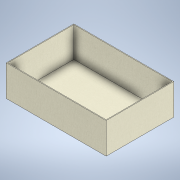
# Autodesk Inventor part: Box_Base
Saved by Autodesk Inventor 2021 (Build 250183000, 183)
## iProperties
Created: 2023-03-16
Part Number: Box_Base
Material: Paper
Document SubType Name: Modeling
Designer: Bradley
Density: 0.93 g/cm^3
Appearance: Cardboard - Chipboard
Author: Bradley
Autodesk Inventor part; units mm, degrees
ref_plane "YZ Plane" through (0, 0, 0) normal (1, 0, 0) x (0, 1, 0)
ref_plane "XZ Plane" through (0, 0, 0) normal (0, 1, 0) x (-1, 0, 0)
ref_plane "XY Plane" through (0, 0, 0) normal (0, 0, 1) x (1, 0, 0)
sketch "Sketch1" plane through (0, 0, 0) normal (0, 1, 0) x (-1, 0, 0)
  line L0 (-212.725, 142.875) -> (212.725, 142.875)
  line L1 (212.725, 142.875) -> (212.725, -142.875)
  line L2 (212.725, -142.875) -> (-212.725, -142.875)
  line L3 (-212.725, -142.875) -> (-212.725, 142.875)
  line L4 (-212.725, 142.875) -> (212.725, -142.875) construction
  line L5 (212.725, 142.875) -> (-212.725, -142.875) construction
  line L6 (-215.9, -146.05) -> (215.9, -146.05)
  line L7 (215.9, -146.05) -> (215.9, 146.05)
  line L8 (215.9, 146.05) -> (-215.9, 146.05)
  line L9 (-215.9, 146.05) -> (-215.9, -146.05)
  point P0 (0, 0)
  dimension "d0" = 425.45
  dimension "d1" = 285.75
  dimension "d2" = 3.175
  constraints: 20 end point, 4 parallel, 2 midpoint, 2 perpendicular, 1 horizontal, 3 other
  measures "d0" distance of L1.end L2.end
  measures "d1" distance of L2.end L0.start
  measures "d2" distance between parallel lines of L2 L6
extrude "Extrusion1" add sketch "Sketch1" against normal blind 3.175 contours L0 L1 L2 L3 | L9 L8 L7 L6
extrude "Extrusion2" add sketch "Sketch1" along normal blind 130.175
body "Solid1"
